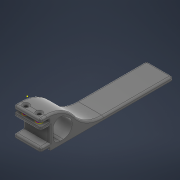
# Autodesk Inventor part: sensorbar
Saved by Autodesk Inventor 2022 (Build 260153000, 153)
## iProperties
Created: 2021-10-11
Part Number: sensorbar
Material: ABS プラスチック
Document SubType Name: Modeling
Designer: shiok
Density: 1.06 g/cm^3
Appearance: 滑らか - 白
Author: shiok
Autodesk Inventor part; units mm, degrees
ref_plane "YZ Plane" through (0, 0, 0) normal (1, 0, 0) x (0, 1, 0)
ref_plane "XZ Plane" through (0, 0, 0) normal (0, 1, 0) x (-1, 0, 0)
ref_plane "XY Plane" through (0, 0, 0) normal (0, 0, 1) x (1, 0, 0)
sketch "スケッチ1" plane through (0, 0, 0) normal (0, 1, 0) x (-1, 0, 0)
  line L0 (-4.0796, 6.5058) -> (-19.0796, 6.5058)
  line L1 (-19.0796, 6.5058) -> (-19.0796, -63.4942)
  line L2 (-19.0796, -63.4942) -> (-4.0796, -63.4942)
  line L3 (-4.0796, -63.4942) -> (-4.0796, 6.5058)
  dimension "d0" = 15
  dimension "d1" = 70
  constraints: 8 end point, 2 parallel, 1 horizontal, 1 perpendicular
  measures "d0" distance of L2.end L1.end
  measures "d1" distance of L1.end L0.end
extrude "押し出し1" add sketch "スケッチ1" along normal blind 2
sketch "スケッチ3" plane through (19.0796, 0, 6.5058) normal (1, 0, 0) x (0, 0, -1)
  line L0 (0, 0) -> (0, 2) projected
  line L1 (0, 2) -> (-5, 2)
  line L2 (-5, 2) -> (-5, 4)
  line L3 (-5, 4) -> (0, 4)
  line L4 (0, 4) -> (0, 12.1)
  line L5 (0, 12.1) -> (-5, 12.1)
  line L6 (-5, 12.1) -> (-5, 14.1)
  line L7 (-5, 14.1) -> (0, 14.1)
  line L8 (0, 14.1) -> (0, 16.1)
  line L9 (0, 16.1) -> (-5, 16.1)
  line L10 (-5, 16.1) -> (-5, 18.1)
  line L11 (-5, 18.1) -> (10, 18.1)
  line L12 (10, 18.1) -> (19.2953, 2)
  line L13 (0, 2) -> (70, 2) projected
  line L14 (19.2953, 2) -> (0, 2)
  line L15 (16.9859, 2) -> (8.8453, 16.1)
  line L16 (8.8453, 16.1) -> (2, 16.1)
  line L17 (2, 16.1) -> (2, 16.6)
  line L18 (2, 16.6) -> (2, 2)
  point P0 (2, 2)
  point P1 (16.9859, 2)
  point P2 (2, 16.1)
  dimension "d8" = 2
  dimension "d9" = 5
  dimension "d10" = 60
  dimension "d11" = 15
  dimension "d12" = 2
  dimension "d13" = 2
  dimension "d58" = 14.1
  constraints: 34 end point, 9 point on line, 7 perpendicular, 4 collinear, 1 horizontal, 1 other
  measures "d8" distance of L1.end L2.end
  measures "d9" distance of L2.end L3.end
  measures "d10" angle of L14 L12
  measures "d11" distance of L10.end L11.end
  measures "d12" distance between parallel lines of L12 L15
  measures "d13" distance between parallel lines of L4 L18
  measures "d58" distance between parallel lines of L11 L3
extrude "押し出し2" add sketch "スケッチ3" against normal up to surface (15 mm away) contours L1 L2 L3 L4 L5 L6 L7 L8 L9 L10 L11 L12 L13 L15 L16 L18
sketch "スケッチ4" plane through (0, 0, 0) normal (0, -1, 0) x (1, 0, 0)
  line L0 (4.0796, 6.5058) -> (19.0796, 6.5058) projected
  line L1 (4.0796, -3.4942) -> (19.0796, -3.4942) projected
  arc A0 (4.0796, 6.5058) -> (19.0796, 6.5058) centre (11.5796, 68.5542) ccw
  point P0 (0, 0)
  dimension "d17" = 62.5
  constraints: 2 point on circle, 1 centre point
  measures "d17" radius of A0
extrude "押し出し3" cut sketch "スケッチ4" against normal up to surface (2 mm away)
sketch "スケッチ5" plane through (0, 0, 0) normal (0, -1, 0) x (1, 0, 0)
  arc A0 (4.0796, 6.5058) -> (19.0796, 6.5058) centre (11.5796, 68.5542) ccw projected
  line L0 (19.0796, 6.5058) -> (19.0796, 11.5058) projected
  arc A1 (4.0796, 6.5058) -> (19.0796, 6.5058) centre (11.5796, 68.5542) ccw
  line L1 (4.0796, -3.4942) -> (4.0796, 11.5058) projected
  line L2 (4.0796, 6.5058) -> (4.0796, 11.5058)
  line L3 (4.0796, 11.5058) -> (19.0796, 11.5058)
  line L4 (19.0796, 11.5058) -> (19.0796, 6.5058)
  point P0 (0, 0)
  point P1 (4.0796, -10.6074)
  dimension "d20" = 62.5
  constraints: 6 end point, 2 point on circle, 1 centre point, 1 parallel
  measures "d20" radius of A1
extrude "押し出し4" cut sketch "スケッチ5" against normal up to surface (2 mm away) from surface at -14.1
fillet "フィレット5" radius 20 1 edges at (11.5796, 16.1, -2.3395)
fillet "フィレット6" radius 20 1 edges at (11.5796, 18.1, -3.4942)
fillet "フィレット7" radius 20 1 edges at (11.5796, 2, -12.7895)
fillet "フィレット8" radius 5 1 edges at (11.5796, 2, -10.4801)
fillet "フィレット9" radius 4 2 edges at (11.5796, 16.1, 4.5058) (11.5796, 2, 4.5058)
fillet "フィレット10" radius 1 8 edges at (4.0796, 4.1254, -15.0497) (4.0796, 15.9746, -0.9193) (4.0796, 18.1, 9.7794) (4.0796, 2, -43.758) (19.0796, 4.1254, -15.0497) (19.0796, 15.9746, -0.9193) (19.0796, 18.1, 9.7794) (19.0796, 2, -43.758)
fillet "フィレット12" radius 1 16 edges at (11.5796, 0, 6.0542) (4.3725, 17.8071, 11.5058) (4.0796, 16.6, 11.5058) (18.7867, 17.8071, 11.5058) (19.0796, 16.6, 11.5058) (11.5796, 18.1, 11.5058) (11.5796, 12.1, 11.5058) (4.0796, 13.1, 11.5058) (19.0796, 13.1, 11.5058) (4.0796, 4, 9.0058) (19.0796, 4, 9.0058) (4.0796, 12.1, 9.0058) (19.0796, 12.1, 9.0058) (4.0796, 3, 11.5058) (19.0796, 3, 11.5058) (11.5796, 4, 11.5058)
fillet "フィレット14" radius 1 5 edges at (18.7867, 1.7071, -63.4942) (11.5796, 2, -63.4942) (4.3725, 1.7071, -63.4942) (4.0796, 0.5, -63.4942) (19.0796, 0.5, -63.4942)
sketch "スケッチ6" plane through (5.0796, 18.1, 8.0529) normal (0, 1, 0) x (1, 0, 0)
  arc A0 (-1, -2.453) -> (0, -3.453) centre (0, -2.453) ccw projected
  line L0 (13, -3.453) -> (0, -3.453) projected
  arc A1 (13, -3.453) -> (14, -2.453) centre (13, -2.453) ccw projected
  line L1 (14, 1.547) -> (14, -2.453) projected
  arc A2 (14, 1.547) -> (-1, 1.547) centre (6.5, -60.5014) ccw projected
  line L2 (-1, 1.547) -> (-1, -2.453) projected
  line L3 (2.75, -0.453) -> (-1, -0.453) construction
  line L4 (0, 0) -> (13, 0) construction
  line L5 (10.25, -0.453) -> (14, -0.453) construction
  line L6 (14, -2.453) -> (14, 1.547) construction
  line L7 (2.75, -0.453) -> (6.5, -0.453) construction
  line L8 (6.5, -0.453) -> (10.25, -0.453) construction
  constraints: 8 end point, 6 collinear, 2 midpoint, 1 coincident
hole "穴1" at (7.8296, 18.1, 8.5058) at (15.3296, 18.1, 8.5058) direction (0, -1, 0) diameter 1.8 depth 2 tip angle 118 countersink diameter 3.6 countersink angle 90 clearance for "Countersunk Flat Head Screw ISO 2009/7046" size "M1.6" standard "ISO"
sketch "スケッチ8" plane through (11.5796, 14.1, 68.5542) normal (0, 1, 0) x (1, 0, 0)
  arc A0 (-5.1274, 60.5014) -> (-2.3726, 60.5014) centre (-3.75, 60.0484) ccw projected
  arc A1 (2.3726, 60.5014) -> (5.1274, 60.5014) centre (3.75, 60.0484) ccw projected
  arc A2 (-5.4921, 60.5014) -> (-2.0079, 60.5014) centre (-3.75, 60.0484) ccw projected
  arc A3 (2.0079, 60.5014) -> (5.4921, 60.5014) centre (3.75, 60.0484) ccw projected
  point P0 (-11.5796, 68.5542)
  constraints: 2 coincident
sketch "スケッチ9" plane through (11.5796, 2, 68.5542) normal (0, -1, 0) x (1, 0, 0)
  circle A0 centre (3.75, -60.0484) radius 0.9 projected
  circle A1 centre (-3.75, -60.0484) radius 0.9 projected
  point P0 (-11.5796, -68.5542)
  point P1 (3.75, -60.0484)
  point P2 (-3.75, -60.0484)
  constraints: 2 coincident
fillet "フィレット15" radius 1 2 edges at (4.0796, 8.05, 6.5058) (19.0796, 8.05, 6.5058)
